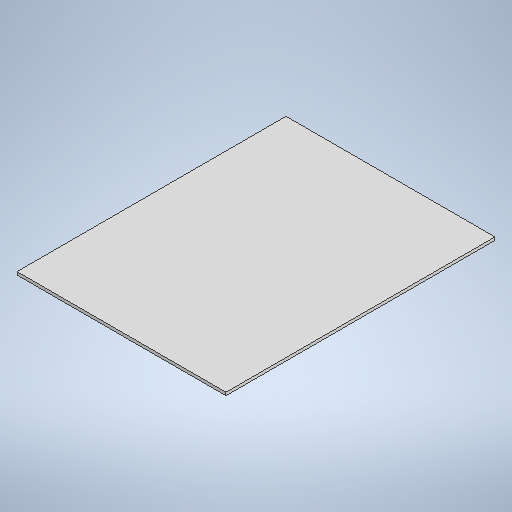
# Autodesk Inventor part: base
Saved by Autodesk Inventor 2025.1 (Build 291241000, 241)
## iProperties
Created: 2025-11-11
Part Number: base
Material: Generic
Document SubType Name: Modeling
Designer: mukund
Density: 1 g/cm^3
Appearance: Default
Author: mukund
Autodesk Inventor part; units mm, degrees
ref_plane "YZ Plane" through (0, 0, 0) normal (1, 0, 0) x (0, 1, 0)
ref_plane "XZ Plane" through (0, 0, 0) normal (0, 1, 0) x (-1, 0, 0)
ref_plane "XY Plane" through (0, 0, 0) normal (0, 0, 1) x (1, 0, 0)
sketch "Sketch1" plane through (0, 0, 0) normal (0, 1, 0) x (-1, 0, 0)
  line L0 (-174, 224) -> (174, 224)
  line L1 (174, 224) -> (174, -224)
  line L2 (174, -224) -> (-174, -224)
  line L3 (-174, -224) -> (-174, 224)
  line L4 (-174, 224) -> (174, -224) construction
  line L5 (174, 224) -> (-174, -224) construction
  point P0 (0, 0)
  dimension "d0" = 348
  dimension "d1" = 448
  constraints: 12 end point, 2 midpoint, 2 parallel, 1 horizontal, 1 perpendicular
  measures "d0" distance of L1.end L2.end
  measures "d1" distance of L0.end L1.end
extrude "Extrusion1" add sketch "Sketch1" along normal blind 5
body "Solid1"
